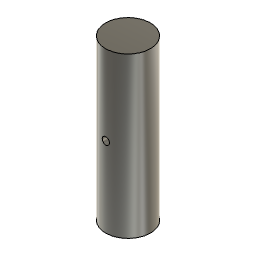
cow-stepper-shaft-mkII (Autodesk Fusion 360 design; units mm, degrees)
Autodesk Fusion 360 part; units mm, degrees
sketch "Sketch1" plane through (0, 0, 0) normal (0, 0, 1) x (1, 0, 0) in component "Shaft"
  circle A0 centre (0, 0) radius 7
  dimension "d4" = 14
  constraint coincident A0.centre origin
  measures "d4" diameter of A0
extrude "Extrude1" add sketch "Sketch1" along normal blind 50 in component "Shaft"
sketch "Sketch2" plane through (0, 0, 0) normal (0, 0, 1) x (1, 0, 0) in component "Shaft"
  circle A0 centre (0, 0) radius 2.6
  line L0 (1.7, 2.6) -> (-1.7, 2.6)
  line L1 (-1.7, 2.6) -> (-1.7, -2.6)
  line L2 (-1.7, -2.6) -> (1.7, -2.6)
  line L3 (1.7, -2.6) -> (1.7, 2.6)
  line L4 (1.7, 2.6) -> (-1.7, -2.6) construction
  line L5 (-1.7, 2.6) -> (1.7, -2.6) construction
  dimension "d8" = 5.2
  dimension "d9" = 3.4
  dimension "d10" = 5.2
  constraint coincident A0.centre origin
  constraint horizontal L0
  constraint perpendicular L0 L1
  constraint parallel L0 L2
  constraint parallel L1 L3
  constraint coincident L4 A0.centre
  constraint coincident L5 A0.centre
  measures "d8" diameter of A0
  measures "d9" distance of L1.end L2.end
  measures "d10" distance of L0.end L1.end
extrude "Extrude2" cut sketch "Sketch2" along normal blind 6 contours A0 L1 L3 in component "Shaft"
sketch "Sketch3" plane through (0, 0, 0) normal (0, 1, 0) x (1, 0, 0) in component "Shaft"
  line L0 (-7, -50) -> (7, -50)
  line L1 (0, 0) -> (0, -50) construction
  circle A0 centre (0, -25) radius 1.125
  dimension "d15" = 50
  dimension "d16" = 2.25
  constraint coincident L1.start origin
  constraint perpendicular L0 L1
  constraint midpoint L1 A0.centre
  measures "d15" distance of L1.start L1.end
  measures "d16" diameter of A0
extrude "Extrude3" cut sketch "Sketch3" along normal blind 7 and the other way blind 7 in component "Shaft"
component "Shaft" placed x (1, 0, 0) y (0, 1, 0) z (0, 0, 1) at (0, 0, 0)
equation "shaftOuterDiameter = 14 mm"
equation "shaftInnerDiameter = 5.2 mm"
equation "shaftInnerSmallDiameter = 3.4 mm"
equation "d4 = shaftOuterDiameter"
equation "shaftHeight = 50 mm"
equation "d6 = shaftHeight"
equation "d8 = shaftInnerDiameter"
equation "d9 = shaftInnerSmallDiameter"
equation "d10 = shaftInnerDiameter"
equation "shaftSmallDepth = 6 mm"
equation "d12 = shaftSmallDepth"
equation "shaftDrillHole = 2.25 mm"
equation "d15 = shaftHeight"
equation "d16 = shaftDrillHole"
equation "d17 = shaftOuterDiameter / 2"
equation "d19 = shaftOuterDiameter / 2"
named bodies: "baseShaft"
